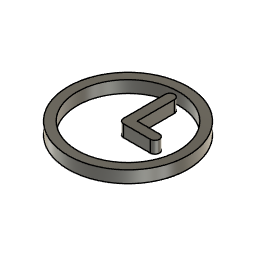
Clock (Autodesk Fusion 360 design; units mm, degrees)
Autodesk Fusion 360 part; units mm, degrees
sketch "スケッチ1" plane through (0, 0, 0) normal (0, 0, 1) x (1, 0, 0)
  line L0 (38.5, 38.5) -> (38.5, 350)
  arc A0 (38.5, 350) -> (-38.5, 350) centre (0, 350) ccw
  line L1 (-38.5, 350) -> (-38.5, 0)
  arc A1 (-38.5, 0) -> (0, -38.5) centre (0, 0) ccw
  line L2 (0, 0) -> (0, 350) construction
  line L3 (0, -38.5) -> (225, -38.5)
  arc A2 (225, -38.5) -> (225, 38.5) centre (225, 0) ccw
  line L4 (225, 38.5) -> (38.5, 38.5)
  arc A3 (-38.5, 0) -> (0, -38.5) centre (0, 0) ccw
  line L5 (0, 0) -> (225, 0) construction
  circle A4 centre (0, 0) radius 425
  circle A5 centre (0, 0) radius 500
  dimension "d1" = 77
  dimension "d2" = 225
  dimension "d3" = 350
  dimension "d4" = 75
  dimension "d5" = 1000
  constraint tangent L0 A0
  constraint tangent A0 L1
  constraint parallel L0 L1
  constraint tangent L1 A1
  constraint tangent L0 A1
  constraint vertical L2
  constraint coincident A1.centre L2.start
  constraint tangent L3 A2
  constraint tangent A2 L4
  constraint parallel L3 L4
  constraint tangent L4 A3
  constraint tangent L3 A3
  constraint perpendicular L0 L5
  constraint concentric A1 A5
  measures "d1" distance of L3.end A2.end
  measures "d2" distance of A1.centre A2.centre
  measures "d3" distance of A1.centre A0.centre
  measures "d4" distance of A4 A5
  measures "d5" diameter of A5
extrude "押し出し1" add sketch "スケッチ1" along normal blind 100 makes body 1 at (497.5154, -49.7839, 33.3333) makes body 2 at (-12.8333, 129.5, 0)
